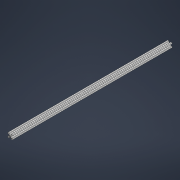
# Autodesk Inventor part: 20x20x100 Aluminium VSlot Extrustion
Saved by Autodesk Inventor 2022 (Build 260153000, 153)
## iProperties
Created: 2022-12-27
Part Number: 20x20x100 Aluminium VSlot Extrustion
Material: Generic
Document SubType Name: Modeling
Designer: Gaming
Density: 1 g/cm^3
Appearance: Default
Author: Gaming
Autodesk Inventor part; units mm, degrees
ref_plane "YZ Plane" through (0, 0, 0) normal (1, 0, 0) x (0, 1, 0)
ref_plane "XZ Plane" through (0, 0, 0) normal (0, 1, 0) x (-1, 0, 0)
ref_plane "XY Plane" through (0, 0, 0) normal (0, 0, 1) x (1, 0, 0)
sketch "Sketch1" plane through (0, 0, 0) normal (0, 0, 1) x (1, 0, 0)
  line L0 (-5, 10) -> (-3.5, 8)
  line L1 (-3.5, 8) -> (-5.5, 8)
  line L2 (5.5, 8) -> (3.5, 8)
  line L3 (3.5, 8) -> (5, 10)
  line L4 (-5.5, 8) -> (-5.5, 6)
  line L5 (5.5, 8) -> (5.5, 6)
  line L6 (-5.5, 6) -> (-2.5, 3)
  line L7 (5.5, 6) -> (2.5, 3)
  line L8 (-2.5, 3) -> (2.5, 3)
  line L9 (-10, 10) -> (-5, 10)
  line L10 (5, 10) -> (10, 10)
  line L11 (3, 2.5) -> (3, -2.5)
  line L12 (3, -2.5) -> (6, -5.5)
  line L13 (6, -5.5) -> (8, -5.5)
  line L14 (8, -5.5) -> (8, -3.5)
  line L15 (8, -3.5) -> (10, -5)
  line L16 (3, 2.5) -> (6, 5.5)
  line L17 (6, 5.5) -> (8, 5.5)
  line L18 (8, 5.5) -> (8, 3.5)
  line L19 (8, 3.5) -> (10, 5)
  line L20 (10, 10) -> (10, 5)
  line L21 (10, -5) -> (10, -10)
  line L22 (-10, 5) -> (-8, 3.5)
  line L23 (-8, 3.5) -> (-8, 5.5)
  line L24 (-8, -5.5) -> (-8, -3.5)
  line L25 (-8, -3.5) -> (-10, -5)
  line L26 (-8, 5.5) -> (-6, 5.5)
  line L27 (-8, -5.5) -> (-6, -5.5)
  line L28 (-6, 5.5) -> (-3, 2.5)
  line L29 (-6, -5.5) -> (-3, -2.5)
  line L30 (-3, 2.5) -> (-3, -2.5)
  line L31 (-10, 10) -> (-10, 5)
  line L32 (-10, -5) -> (-10, -10)
  line L33 (-2.5, -3) -> (2.5, -3)
  line L34 (2.5, -3) -> (5.5, -6)
  line L35 (5.5, -6) -> (5.5, -8)
  line L36 (5.5, -8) -> (3.5, -8)
  line L37 (3.5, -8) -> (5, -10)
  line L38 (-2.5, -3) -> (-5.5, -6)
  line L39 (-5.5, -6) -> (-5.5, -8)
  line L40 (-5.5, -8) -> (-3.5, -8)
  line L41 (-3.5, -8) -> (-5, -10)
  line L42 (-10, -10) -> (-5, -10)
  line L43 (5, -10) -> (10, -10)
  point P0 (0, 0)
  point P1 (0, 0)
  point P2 (0, 0)
  dimension "d0" = 20
  dimension "d1" = 20
  dimension "d3" = 2
  dimension "d4" = 2
  dimension "d6" = 1.5
  dimension "d7" = 2
  dimension "d8" = 2
  dimension "d9" = 3
  dimension "d11" = 3
  dimension "d12" = 3
  dimension "d13" = 5
  dimension "d22" = 5
  dimension "d24" = 3
  dimension "d25" = 3
  dimension "d26" = 2
  dimension "d27" = 5
  dimension "d28" = 2
  dimension "d29" = 2
  dimension "d30" = 1.5
  dimension "d31" = 3
  dimension "d32" = 5
  dimension "d33" = 5
  dimension "d35" = 5
  dimension "d36" = 5
  dimension "d37" = 5
  dimension "d38" = 5
  dimension "d40" = 3
  dimension "d41" = 3
  dimension "d42" = 2
  dimension "d43" = 2
  dimension "d48" = 3
  dimension "d49" = 3
  dimension "d50" = 3
  dimension "d51" = 3
  dimension "d52" = 0.5
  dimension "d53" = 0.5
  dimension "d54" = 0.5
  dimension "d55" = 0.5
  dimension "d56" = 0.5
  constraints: 88 end point, 25 equal length, 13 perpendicular, 4 coincident, 4 horizontal, 4 vertical, 1 horizontal alignment
  measures "d0" distance of L9.start L10.end
  measures "d1" distance of L10.end L21.end
  measures "d3" vertical distance of L0.end L0.start
  measures "d4" vertical distance of L3.end L2.end
  measures "d6" horizontal distance of L0.end L0.start
  measures "d7" distance of L0.end L1.end
  measures "d8" distance of L1.end L4.end
  measures "d9" horizontal distance of L6.end L4.end
  measures "d11" horizontal distance of L6.end L4.end
  measures "d12" horizontal distance of L5.end L7.end
  measures "d13" distance of L7.end L6.end
  measures "d22" distance of L11.start L11.end
  measures "d24" horizontal distance of L11.end L12.end
  measures "d25" horizontal distance of L12.end L11.end
  measures "d26" distance of L13.end L12.end
  measures "d27" distance of L9.start L0.start
  measures "d28" distance of L13.end L14.end
  measures "d29" horizontal distance of L15.end L14.end
  measures "d30" vertical distance of L14.end L15.end
  measures "d31" horizontal distance of L11.start L16.end
  measures "d32" distance of L21.end L15.end
  measures "d33" distance of L10.end L19.end
  measures "d35" distance of L37.end L21.end
  measures "d36" distance of L9.start L22.start
  measures "d37" distance of L32.end L42.end
  measures "d38" distance of L32.start L32.end
  measures "d40" horizontal distance of L38.start L39.start
  measures "d41" horizontal distance of L29.start L29.end
  measures "d42" vertical distance of L41.start L42.end
  measures "d43" horizontal distance of L24.end L32.start
  measures "d48" distance from line of L11 point (0, 0)
  measures "d49" distance from line of L30 point (0, 0)
  measures "d50" distance from line of L8 point (0, 0)
  measures "d51" distance from line of L33 point (0, 0)
  measures "d52" horizontal distance of L29.end L38.start
  measures "d53" horizontal distance of L29.end L38.start
  measures "d54" horizontal distance of L11.end L34.start
  measures "d55" horizontal distance of L11.end L34.start
  measures "d56" horizontal distance of L7.end L11.start
extrude "Extrusion3" add sketch "Sketch1" along normal blind 740
sketch "Sketch3" plane through (0, 0, 0) normal (0, 0, -1) x (-1, 0, 0)
  circle A0 centre (0, 0) radius 2
  dimension "d59" = 4
  constraints: 1 centre point, 1 coincident
  measures "d59" diameter of A0
extrude "Extrusion4" cut sketch "Sketch3" against normal through all
body "Solid2"
